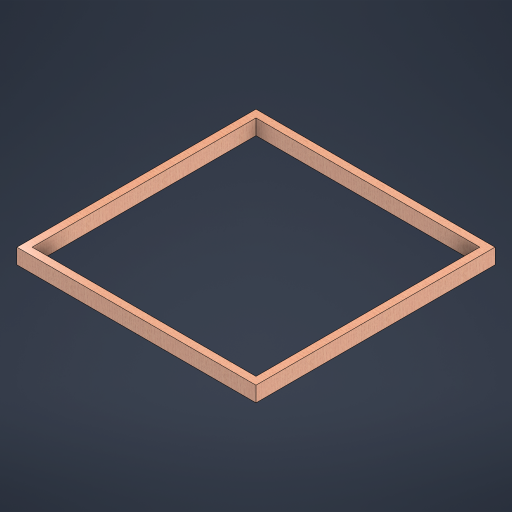
# Autodesk Inventor part: 200554
Saved by Autodesk Inventor 2023.1 (Build 271208000, 208)
## iProperties
Created: 2023-01-06
Part Number: 200554
Material: Wood (Oak)
Document SubType Name: Modeling
Designer: Byron Robotics
Mass: 3013.91 g
Surface Area: 4683.86 cm^2
Volume: 3965.67 cm^3
Density: 0.76 g/cm^3
Appearance: White Oak - Natural Medium Gloss
Author: Byron Robotics
Autodesk Inventor part; units mm, degrees
ref_plane "YZ Plane" through (0, 0, 0) normal (1, 0, 0) x (0, 1, 0)
ref_plane "XZ Plane" through (0, 0, 0) normal (0, 1, 0) x (-1, 0, 0)
ref_plane "XY Plane" through (0, 0, 0) normal (0, 0, 1) x (1, 0, 0)
sketch "Sketch1" plane through (0, 0, 0) normal (0, 1, 0) x (-1, 0, 0)
  line L0 (0, 0) -> (742.95, 0)
  line L1 (742.95, 0) -> (742.95, 742.95)
  line L2 (742.95, 742.95) -> (0, 742.95)
  line L3 (0, 742.95) -> (0, 0)
  line L4 (0, 742.95) -> (742.95, 0) construction
  line L5 (0, 0) -> (742.95, 742.95) construction
  line L6 (768.35, -25.4) -> (-25.4, -25.4)
  line L7 (-25.4, -25.4) -> (-25.4, 768.35)
  line L8 (-25.4, 768.35) -> (768.35, 768.35)
  line L9 (768.35, 768.35) -> (768.35, -25.4)
  line L10 (768.35, -25.4) -> (-25.4, 768.35) construction
  line L11 (-25.4, -25.4) -> (768.35, 768.35) construction
  point P0 (371.475, 371.475)
  point P1 (-25.4, 371.475)
  dimension "d0" = 742.95
  dimension "d2" = 25.4
  dimension "d3" = 25.4
  constraints: 24 end point, 4 midpoint, 4 parallel, 4 perpendicular, 2 horizontal
  measures "d0" distance of L1.end L2.end
  measures "d2" distance from line of L3 point (-25.4, 371.475)
  measures "d3" distance between parallel lines of L2 L8
extrude "Extrusion1" add sketch "Sketch1" along normal blind 50.8
body "Solid1"
